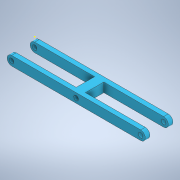
# Autodesk Inventor part: Joint 1
Saved by Autodesk Inventor 2021 (Build 250183000, 183)
## iProperties
Created: 2021-04-01
Part Number: Joint 1
Material: Generic
Document SubType Name: Modeling
Designer: Darek
Density: 1 g/cm^3
Appearance: Anodized - Light Gray
Mass: 15.8037 g
Surface Area: 102.174 cm^2
Volume: 15.8037 cm^3
Author: Darek
Autodesk Inventor part; units mm, degrees
ref_plane "YZ Plane" through (0, 0, 0) normal (1, 0, 0) x (0, 1, 0)
ref_plane "XZ Plane" through (0, 0, 0) normal (0, 1, 0) x (-1, 0, 0)
ref_plane "XY Plane" through (0, 0, 0) normal (0, 0, 1) x (1, 0, 0)
sketch "Sketch1" plane through (0, 0, 0) normal (0, 0, 1) x (1, 0, 0)
  line L0 (0, 0) -> (150, 0)
  line L1 (150, 0) -> (150, 10)
  line L2 (150, 10) -> (0, 10)
  line L3 (0, 10) -> (0, 0)
  circle A0 centre (5, 5) radius 2.5
  circle A1 centre (145, 5) radius 2.5
  dimension "d0" = 5
  dimension "d1" = 5
  dimension "d2" = 10
  dimension "d3" = 5
  dimension "d4" = 150
  dimension "d5" = 5
  dimension "d6" = 5
  dimension "d7" = 5
  constraints: 8 end point, 3 perpendicular, 2 centre point, 1 horizontal
  measures "d0" diameter of A0
  measures "d1" distance from line of L0 A0.centre
  measures "d2" distance between parallel lines of L0 L2
  measures "d3" distance from line of L3 A0.centre
  measures "d4" distance between parallel lines of L3 L1
  measures "d5" distance from line of L2 A1.centre
  measures "d6" distance from line of L1 A1.centre
  measures "d7" diameter of A1
extrude "Extrusion1" add sketch "Sketch1" along normal blind 30
sketch "Sketch2" plane through (0, 10, 0) normal (0, 1, 0) x (1, 0, 0)
  point P0 (0, 0)
sketch "Sketch3" plane through (0, 10, 0) normal (0, 1, 0) x (1, 0, 0)
  line L0 (0, 0) -> (0, -30) projected
  line L1 (0, -25) -> (70, -25)
  line L2 (70, -25) -> (70, -5)
  line L3 (70, -5) -> (0, -5)
  line L4 (0, -5) -> (0, -25)
  line L5 (150, 0) -> (150, -30) projected
  line L6 (150, -25) -> (80, -25)
  line L7 (80, -25) -> (80, -5)
  line L8 (80, -5) -> (150, -5)
  line L9 (150, -5) -> (150, -25)
  line L10 (150, 0) -> (0, 0) projected
  line L11 (150, -30) -> (0, -30) projected
  point P0 (0, -5)
  dimension "d10" = 70
  dimension "d11" = 70
  dimension "d12" = 5
  dimension "d13" = 5
  dimension "d14" = 5
  dimension "d15" = 5
  constraints: 16 end point, 4 parallel, 2 horizontal, 2 perpendicular, 2 point on line
  measures "d10" distance between parallel lines of L2 L0
  measures "d11" distance between parallel lines of L5 L7
  measures "d12" distance between parallel lines of L3 L10
  measures "d13" distance between parallel lines of L11 L1
  measures "d14" distance between parallel lines of L10 L8
  measures "d15" distance between parallel lines of L11 L6
extrude "Extrusion2" cut sketch "Sketch3" against normal blind 10 contours L3 L2 L1 L0 | L5 L6 L7 L8
fillet "Fillet1" radius 5 8 edges at (0, 10, 27.5) (150, 10, 27.5) (150, 10, 2.5) (0, 10, 2.5) (150, 0, 27.5) (150, 0, 2.5) (0, 0, 27.5) (0, 0, 2.5)
sketch "Sketch4" plane through (0, 0, 30) normal (0, 0, 1) x (1, 0, 0)
  circle A0 centre (75, 5) radius 2.5
  line L0 (5, 0) -> (145, 0) projected
  circle A1 centre (5, 5) radius 2.5 projected
  point P0 (0, 0)
  dimension "d19" = 5
  dimension "d20" = 5
  dimension "d21" = 70
  constraints: 1 centre point
  measures "d19" diameter of A0
  measures "d20" distance from line of L0 A0.centre
  measures "d21" distance of A1.centre A0.centre
extrude "Extrusion3" cut sketch "Sketch4" against normal blind 30 contours A0
body "Solid1"
